Autodesk Inventor part; units mm, degrees
(part 2 of 2)
ref_plane "to_L_Winkel_1_YZ" through (-98.75, 0, -61.025) normal (0, 0, -1) x (0, -1, 0)
ref_plane "to_L_Winkel_1_ZX" through (-98.75, 0, -61.025) normal (0, -1, 0) x (-1, 0, 0)
ref_plane "to_MP_XY" through (0, 0, -61.125) normal (0, 0, -1) x (1, 0, 0)
ref_plane "to_MP_YZ" through (0, 0, -61.125) normal (1, 0, 0) x (0, -1, 0)
ref_plane "to_MP_ZX" through (0, 0, -61.125) normal (0, -1, 0) x (0, 0, -1)
body "Solid1"
